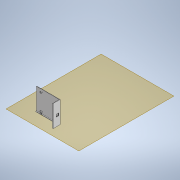
# Autodesk Inventor part: Rambo Case
Saved by Autodesk Inventor 2020 (Build 240168000, 168)
## iProperties
Created: 2019-12-13
Part Number: Rambo Case
Material: Generic
Document SubType Name: Modeling
Designer: pepd9
Density: 1 g/cm^3
Appearance: Default
Author: pepd9
Autodesk Inventor part; units mm, degrees
ref_plane "YZ Plane" through (0, 0, 0) normal (1, 0, 0) x (0, 1, 0)
ref_plane "XZ Plane" through (0, 0, 0) normal (0, 1, 0) x (-1, 0, 0)
ref_plane "XY Plane" through (0, 0, 0) normal (0, 0, 1) x (1, 0, 0)
ref_plane "Work Plane1" through (-3.5096, -12.3151, -160.6613) normal (0, 1, 0) x (0, 0, 1)
sketch "Sketch1" plane through (-3.5096, -12.3151, -160.6613) normal (0, 1, 0) x (0, 0, 1)
  circle A0 centre (196, -5.2) radius 1.1 projected
  circle A1 centre (196, -80) radius 1.1 projected
  circle A2 centre (196, -5.2) radius 3
  circle A3 centre (196, -80) radius 3
  point P0 (160.6613, 3.5096)
  dimension "d0" = 6
  dimension "d1" = 6
  constraints: 2 centre point, 2 coincident
  measures "d0" diameter of A2
  measures "d1" diameter of A3
extrude "Extrusion1" add sketch "Sketch1" along normal blind 5
ref_plane "Work Plane2" through (-3.5096, -12.3151, -160.6613) normal (0, 1, 0) x (0, 0, 1)
sketch "Sketch2" plane through (-3.5096, -12.3151, -160.6613) normal (0, 1, 0) x (0, 0, 1)
  line L0 (193, 21.1576) -> (199, 21.1576)
  line L1 (199, 21.1576) -> (199, -108.8424)
  line L2 (199, -108.8424) -> (193, -108.8424)
  line L3 (193, -108.8424) -> (193, 21.1576)
  circle A0 centre (196, -5.2) radius 3 projected
  circle A1 centre (196, -80) radius 3 projected
  point P0 (160.6613, 3.5096)
  point P1 (200, 20.1576)
  point P2 (193, -5.2)
  point P3 (193, -80)
  dimension "d4" = 130
  dimension "d5" = 1
  dimension "d8" = 6
  constraints: 8 end point, 2 parallel, 1 horizontal, 1 perpendicular, 1 other
  measures "d4" distance of L2.end L0.start
  measures "d5" distance from line of L0 point (200, 20.158)
  measures "d8" distance of L0.start L0.end
extrude "Extrusion2" add sketch "Sketch2" along normal blind 3 contours L0 L1 A0 L3 | A0 L1 A1 L3 | A1 L1 L2 L3
sketch "Sketch3" plane through (-83.5096, -7.3151, 35.3387) normal (0, 1, 0) x (1, 0, 0)
  circle A0 centre (74.8, 0) radius 3 projected
  circle A1 centre (74.8, 0) radius 1.1 projected
  circle A2 centre (0, 0) radius 3 projected
  circle A3 centre (0, 0) radius 1.1 projected
  line L0 (101.1576, 3) -> (-28.8424, 3) projected
  line L1 (-3, 0) -> (3, 0)
  line L2 (3, 0) -> (3, 3)
  line L3 (3, 3) -> (-3, 3)
  line L4 (-3, 3) -> (-3, 0)
  line L5 (71.8, 0) -> (77.8, 0)
  line L6 (77.8, 0) -> (77.8, 3)
  line L7 (77.8, 3) -> (71.8, 3)
  line L8 (71.8, 3) -> (71.8, 0)
  point P0 (83.5096, 35.3387)
  point P1 (71.8, 3)
  point P2 (74.8, 3)
  point P3 (77.8, 3)
  point P4 (0, 3)
  point P5 (-3, 3)
  constraints: 16 end point, 4 parallel, 3 point on line, 2 horizontal, 2 perpendicular, 4 other
extrude "Extrusion3" add sketch "Sketch3" against normal up to surface (2 mm away) contours L8 L0 A0 | A0 L0 L6 | L4 L0 A2 | A2 L0 L2
sketch "Sketch4" plane through (-3.5096, -9.3151, -160.6613) normal (0, 1, 0) x (1, 0, 0)
  line L0 (-2.2, -193) -> (-2.2, -196) projected
  arc A0 (-5.2, -199) -> (-2.2, -196) centre (-5.2, -196) ccw projected
  line L1 (-5.2, -199) -> (21.1576, -199) projected
  line L2 (21.1576, -199) -> (21.1576, -193) projected
  line L3 (21.1576, -193) -> (-2.2, -193) projected
  line L4 (-8.2, -196) -> (-8.2, -193) projected
  line L5 (-8.2, -193) -> (-77, -193) projected
  line L6 (-77, -193) -> (-77, -196) projected
  arc A1 (-80, -199) -> (-77, -196) centre (-80, -196) ccw projected
  line L7 (-80, -199) -> (-5.2, -199) projected
  arc A2 (-8.2, -196) -> (-5.2, -199) centre (-5.2, -196) ccw projected
  line L8 (-83, -196) -> (-83, -193) projected
  line L9 (-83, -193) -> (-108.8424, -193) projected
  line L10 (-108.8424, -193) -> (-108.8424, -199) projected
  line L11 (-108.8424, -199) -> (-80, -199) projected
  arc A3 (-83, -196) -> (-80, -199) centre (-80, -196) ccw projected
  line L12 (21.1576, -199) -> (21.1576, -193) projected
  line L13 (-108.8424, -193) -> (21.1576, -193)
  line L14 (21.1576, -193) -> (21.1576, -195)
  line L15 (21.1576, -195) -> (-108.8424, -195)
  line L16 (-108.8424, -195) -> (-108.8424, -193)
  point P0 (3.5096, -160.6613)
  point P1 (-2.2, -193)
  point P2 (-8.2, -193)
  point P3 (-83, -193)
  point P4 (-108.8424, -195)
  dimension "d11" = 2
  constraints: 8 end point, 2 parallel, 1 horizontal, 1 perpendicular, 1 point on line
  measures "d11" distance of L13.end L14.end
extrude "Extrusion4" add sketch "Sketch4" along normal blind 120 contours L3 L2 L15 L0 | L0 L15 L4 L13 | L4 L15 L6 L5 | L6 L15 L8 L13 | L8 L15 L10 L9
sketch "Sketch5" plane through (17.648, -12.3151, 32.3387) normal (0, 0, -1) x (-1, 0, 0)
  point P0 (17.648, 12.3151)
  point P1 (29.3576, 5)
  point P2 (23.3576, 5)
  point P3 (104.1576, 5)
  point P4 (98.1576, 5)
sketch "Sketch6" plane through (-80.5096, -9.3151, 34.3387) normal (0, 0, 1) x (1, 0, 0)
  circle A0 centre (93.3476, 10.81) radius 1.5 projected
  circle A1 centre (-3.1724, 10.81) radius 1.5 projected
  circle A2 centre (-3.1724, 106.06) radius 1.5 projected
  circle A3 centre (93.3476, 106.06) radius 1.5 projected
  line L0 (97.5976, 103.6063) -> (93.3476, 101.1525)
  line L1 (93.3476, 101.1525) -> (89.0976, 103.6063)
  line L2 (89.0976, 103.6063) -> (89.0976, 108.5137)
  line L3 (89.0976, 108.5137) -> (93.3476, 110.9675)
  line L4 (93.3476, 110.9675) -> (97.5976, 108.5137)
  line L5 (97.5976, 108.5137) -> (97.5976, 103.6063)
  line L6 (97.5976, 8.3563) -> (93.3476, 5.9025)
  line L7 (93.3476, 5.9025) -> (89.0976, 8.3563)
  line L8 (89.0976, 8.3563) -> (89.0976, 13.2637)
  line L9 (89.0976, 13.2637) -> (93.3476, 15.7175)
  line L10 (93.3476, 15.7175) -> (97.5976, 13.2637)
  line L11 (97.5976, 13.2637) -> (97.5976, 8.3563)
  line L12 (1.0776, 103.6063) -> (-3.1724, 101.1525)
  line L13 (-3.1724, 101.1525) -> (-7.4224, 103.6063)
  line L14 (-7.4224, 103.6063) -> (-7.4224, 108.5137)
  line L15 (-7.4224, 108.5137) -> (-3.1724, 110.9675)
  line L16 (-3.1724, 110.9675) -> (1.0776, 108.5137)
  line L17 (1.0776, 108.5137) -> (1.0776, 103.6063)
  line L18 (1.0776, 8.3563) -> (-3.1724, 5.9025)
  line L19 (-3.1724, 5.9025) -> (-7.4224, 8.3563)
  line L20 (-7.4224, 8.3563) -> (-7.4224, 13.2637)
  line L21 (-7.4224, 13.2637) -> (-3.1724, 15.7175)
  line L22 (-3.1724, 15.7175) -> (1.0776, 13.2637)
  line L23 (1.0776, 13.2637) -> (1.0776, 8.3563)
  point P0 (80.5096, 9.3151)
  point P1 (97.5976, 10.81)
  point P2 (1.0776, 10.81)
  dimension "d14" = 8.5
  dimension "d15" = 8.5
  dimension "d16" = 8.5
  dimension "d17" = 8.5
  constraints: 48 end point, 4 coincident, 2 midpoint, 2 point on line, 2 vertical, 52 other
  measures "d14" distance between parallel lines of L17 L14
  measures "d15" distance between parallel lines of L23 L20
  measures "d16" distance between parallel lines of L2 L5
  measures "d17" distance between parallel lines of L11 L8
ref_plane "Work Plane3" through (-87.492, -2.3151, 39.3387) normal (0, 0, -1) x (0, 1, 0)
extrude "Extrusion5" add sketch "Sketch6" along normal up to surface (5 mm away) contours A0 | A1 | A2 | A3 | L0 L1 L2 L3 L4 L5 | L6 L7 L8 L9 L10 L11 | L12 L13 L14 L15 L16 L17 | L18 L19 L20 L21 L22 L23
sketch "Sketch7" plane through (-87.932, 94.2911, 39.3387) normal (0, 0, 1) x (1, 0, 0)
  circle A0 centre (100.77, 2.4537) radius 1.5 projected
  circle A1 centre (100.77, -92.7963) radius 1.5 projected
  circle A2 centre (4.25, -92.7963) radius 1.5 projected
  circle A3 centre (4.25, 2.4537) radius 1.5 projected
  point P0 (87.932, -94.2911)
hole "Hole1" at (-83.682, 96.7449, 39.3387) at (-83.682, 1.4949, 39.3387) at (12.838, 1.4949, 39.3387) at (12.838, 96.7449, 39.3387) direction (0, 0, -1) diameter 3.4 end through all clearance for "Socket Head Cap Screw" size "M3" standard "Ansi Metric M Profile"
sketch "Sketch8" plane through (17.648, -12.3151, 32.3387) normal (0, 0, -1) x (-1, 0, 0)
  circle A0 centre (4.81, 13.81) radius 1.7 projected
  circle A1 centre (4.81, 109.06) radius 1.7 projected
  circle A2 centre (101.33, 109.06) radius 1.7 projected
  circle A3 centre (101.33, 13.81) radius 1.7 projected
  line L0 (2.06, 15.3977) -> (4.81, 16.9854)
  line L1 (4.81, 16.9854) -> (7.56, 15.3977)
  line L2 (7.56, 15.3977) -> (7.56, 12.2223)
  line L3 (7.56, 12.2223) -> (4.81, 10.6346)
  line L4 (4.81, 10.6346) -> (2.06, 12.2223)
  line L5 (2.06, 12.2223) -> (2.06, 15.3977)
  line L6 (2.06, 110.6477) -> (4.81, 112.2354)
  line L7 (4.81, 112.2354) -> (7.56, 110.6477)
  line L8 (7.56, 110.6477) -> (7.56, 107.4723)
  line L9 (7.56, 107.4723) -> (4.81, 105.8846)
  line L10 (4.81, 105.8846) -> (2.06, 107.4723)
  line L11 (2.06, 107.4723) -> (2.06, 110.6477)
  line L12 (98.58, 110.6477) -> (101.33, 112.2354)
  line L13 (101.33, 112.2354) -> (104.08, 110.6477)
  line L14 (104.08, 110.6477) -> (104.08, 107.4723)
  line L15 (104.08, 107.4723) -> (101.33, 105.8846)
  line L16 (101.33, 105.8846) -> (98.58, 107.4723)
  line L17 (98.58, 107.4723) -> (98.58, 110.6477)
  line L18 (98.58, 15.3977) -> (101.33, 16.9854)
  line L19 (101.33, 16.9854) -> (104.08, 15.3977)
  line L20 (104.08, 15.3977) -> (104.08, 12.2223)
  line L21 (104.08, 12.2223) -> (101.33, 10.6346)
  line L22 (101.33, 10.6346) -> (98.58, 12.2223)
  line L23 (98.58, 12.2223) -> (98.58, 15.3977)
  point P0 (17.648, 12.3151)
  point P1 (98.58, 13.81)
  dimension "d27" = 5.5
  dimension "d28" = 5.5
  dimension "d29" = 5.5
  constraints: 48 end point, 4 coincident, 4 vertical, 1 midpoint, 1 point on line, 52 other
  measures "d27" distance from line of point (98.58, 13.81) L20
  measures "d28" distance between parallel lines of L11 L8
  measures "d29" distance between parallel lines of L2 L5
extrude "Extrusion6" cut sketch "Sketch8" against normal blind 3 contours A1 | L0 L1 L2 L3 L4 L5 | L6 L7 L8 L9 L10 L11 | L12 L13 L14 L15 L16 L17 | L18 L19 L20 L21 L22 L23
sketch "Sketch9" plane through (17.648, -12.3151, 32.3387) normal (0, 0, -1) x (-1, 0, 0)
  line L0 (0, 0) -> (0, 123) projected
  line L1 (0, 0) -> (-2.4, 0)
  line L2 (-2.4, 0) -> (-2.4, 123)
  line L3 (-2.4, 123) -> (0, 123)
  line L4 (0, 123) -> (0, 0)
  point P0 (17.648, 12.3151)
  dimension "d32" = 2.4
  dimension "d33" = 123
  constraints: 8 end point, 2 parallel, 1 horizontal, 1 perpendicular
  measures "d32" distance of L2.end L3.end
  measures "d33" distance of L1.end L2.end
extrude "Extrusion7" add sketch "Sketch9" against normal blind 40
sketch "Sketch10" plane through (20.048, -12.3151, 32.3387) normal (1, 0, 0) x (0, 0, -1)
  arc A0 (-9, 59.85) -> (-9.5, 60.35) centre (-9.5, 59.85) ccw projected
  line L0 (-9.5, 60.35) -> (-19.7, 60.35) projected
  arc A1 (-19.7, 60.35) -> (-20.2, 59.85) centre (-19.7, 59.85) ccw projected
  line L1 (-20.2, 59.85) -> (-20.2, 49.05) projected
  arc A2 (-20.2, 49.05) -> (-19.7, 48.55) centre (-19.7, 49.05) ccw projected
  line L2 (-19.7, 48.55) -> (-9.5, 48.55) projected
  arc A3 (-9.5, 48.55) -> (-9, 49.05) centre (-9.5, 49.05) ccw projected
  line L3 (-9, 49.05) -> (-9, 59.85) projected
  line L4 (-19.7, 60.75) -> (-9.5, 60.75)
  arc A4 (-8.6, 59.85) -> (-9.5, 60.75) centre (-9.5, 59.85) ccw
  line L5 (-8.6, 59.85) -> (-8.6, 49.05)
  arc A5 (-9.5, 48.15) -> (-8.6, 49.05) centre (-9.5, 49.05) ccw
  line L6 (-9.5, 48.15) -> (-19.7, 48.15)
  arc A6 (-20.6, 49.05) -> (-19.7, 48.15) centre (-19.7, 49.05) ccw
  line L7 (-20.6, 49.05) -> (-20.6, 59.85)
  arc A7 (-19.7, 60.75) -> (-20.6, 59.85) centre (-19.7, 59.85) ccw
  point P0 (32.3387, 12.3151)
  dimension "d36" = 0.4
  constraints: 8 end point, 8 point on circle, 4 centre point, 7 other
  measures "d36" distance between parallel lines of L0 L4
extrude "Extrusion8" cut sketch "Sketch10" against normal up to surface (2.4 mm away) contours L3 A3 L2 A2 L1 A1 L0 A0 | L4 A4 L5 A5 L6 A6 L7 A7
chamfer "Chamfer1" distance 1 angle 45 8 edges at (20.048, 42.1349, 40.9387) (20.048, 36.0985, 41.2023) (20.048, 35.8349, 46.9387) (20.048, 36.0985, 52.6751) (20.048, 42.1349, 52.9387) (20.048, 48.1713, 52.6751) (20.048, 48.4349, 46.9387) (20.048, 48.1713, 41.2023)
move faces "Move1" translate (0, 0, 34) faces at (-59.4045, -11.3151, 38.3387)
fillet "Fillet1" radius 3 1 edges at (17.648, -9.3151, 53.3387)
body "Solid1"
